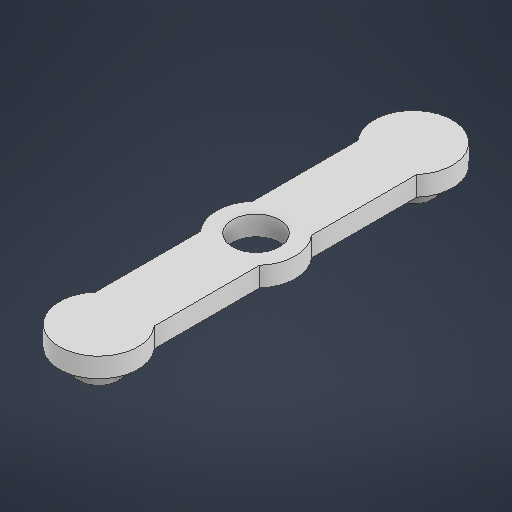
# Autodesk Inventor part: link-split-8ab-2endpins
Saved by Autodesk Inventor 2025.4 (Build 294407000, 407)
## iProperties
Created: 2026-09-15
Part Number: link-split-8ab-2endpins
Material: Generic
Document SubType Name: Modeling
Designer: User
Density: 1 g/cm^3
Appearance: Default
Author: User
Autodesk Inventor part; units mm, degrees
ref_plane "YZ Plane" through (0, 0, 0) normal (1, 0, 0) x (0, 1, 0)
ref_plane "XZ Plane" through (0, 0, 0) normal (0, 1, 0) x (-1, 0, 0)
ref_plane "XY Plane" through (0, 0, 0) normal (0, 0, 1) x (1, 0, 0)
sketch "Sketch1" plane through (0, 0, 0) normal (0, 1, 0) x (-1, 0, 0)
  line L0 (-1.5, -4) -> (1.5, -4)
  line L1 (1.5, -4) -> (1.5, 4)
  line L2 (1.5, 4) -> (-1.5, 4)
  line L3 (-1.5, 4) -> (-1.5, -4)
  line L4 (-1.5, -4) -> (1.5, 4) construction
  line L5 (1.5, -4) -> (-1.5, 4) construction
  circle A0 centre (0, 4) radius 1.2
  circle A1 centre (0, -4) radius 1.2
  circle A2 centre (0, -4) radius 2
  circle A3 centre (0, 4) radius 2
  line L6 (-1.5, 4) -> (1.5, 4)
  line L7 (1.5, 4) -> (1.5, 12)
  line L8 (1.5, 12) -> (-1.5, 12)
  line L9 (-1.5, 12) -> (-1.5, 4)
  circle A4 centre (0, 12) radius 2
  circle A5 centre (0, 12) radius 1.2
  point P0 (0, 0)
  point P1 (-1.5, -2.6771)
  point P2 (1.5, -2.6771)
  point P3 (1.5, 2.6771)
  point P4 (-1.5, 2.6771)
  point P5 (1.5, 10.6771)
  point P6 (-1.5, 10.6771)
  point P7 (-1.5, 5.3229)
  point P8 (1.5, 5.3229)
  dimension "d0" = 3
  dimension "linkPitchA" = 8
  dimension "d3" = 2.4
  dimension "d4" = 4
  dimension "linkPitchB" = 8
  constraints: 20 end point, 6 centre point, 5 midpoint, 5 parallel, 4 equal radius, 3 coincident, 2 horizontal, 2 perpendicular
  measures "d0" distance of L2.end L1.end
  measures "linkPitchA" distance of L1.end L0.end
  measures "d3" diameter of A1
  measures "d4" diameter of A2
  measures "linkPitchB" distance of L7.end L6.end
extrude "Extrusion1" add sketch "Sketch1" along normal blind 1 contours A1 L0 L3 A2 L1 | L0 L1 A2 L3 A1 | A2 L3 A3 L1 | A3 L3 L2 A0 L1 | L1 L7 A3 | L2 A0 L9 A3 L7 | A3 L9 L3 | A3 L9 A4 L7 | A4 L9 L8 A5 L7 | L7 L8 A5 L9 A4
ref_plane "Work Plane2" through (0, 0.5, 0) normal (0, 1, 0) x (1, 0, 0)
sketch "Sketch2" plane through (0, 1, 0) normal (0, 1, 0) x (1, 0, 0)
  line L0 (-1.5, 2.6771) -> (-1.5, -2.6771) projected
  arc A0 (-1.5, -2.6771) -> (-1.5, -5.3229) centre (0, -4) ccw projected
  line L1 (-1.5, -5.3229) -> (-1.5, -10.6771) projected
  arc A1 (-1.5, -10.6771) -> (1.5, -10.6771) centre (0, -12) ccw projected
  line L2 (1.5, -10.6771) -> (1.5, -5.3229) projected
  arc A2 (1.5, -5.3229) -> (1.5, -2.6771) centre (0, -4) ccw projected
  line L3 (1.5, -2.6771) -> (1.5, 2.6771) projected
  arc A3 (1.5, 2.6771) -> (-1.5, 2.6771) centre (0, 4) ccw projected
  circle A4 centre (0, 4) radius 1.2 projected
  circle A5 centre (0, -4) radius 1.2 projected
  circle A6 centre (0, -12) radius 1.2 projected
  circle A7 centre (0, -12) radius 1
  point P0 (0, 0)
  dimension "d22" = 2
  constraints: 1 centre point, 1 coincident
  measures "d22" diameter of A7
extrude "Extrusion2" add sketch "Sketch2" along normal blind 0.5 and the other way blind 1.5 from surface at -0.5 contours A7
sketch "Sketch3" plane through (0, 1, 0) normal (0, 1, 0) x (1, 0, 0)
  line L0 (-1.5, 2.6771) -> (-1.5, -2.6771) projected
  arc A0 (-1.5, -2.6771) -> (-1.5, -5.3229) centre (0, -4) ccw projected
  line L1 (-1.5, -5.3229) -> (-1.5, -10.6771) projected
  arc A1 (-1.5, -10.6771) -> (1.5, -10.6771) centre (0, -12) ccw projected
  line L2 (1.5, -10.6771) -> (1.5, -5.3229) projected
  arc A2 (1.5, -5.3229) -> (1.5, -2.6771) centre (0, -4) ccw projected
  line L3 (1.5, -2.6771) -> (1.5, 2.6771) projected
  arc A3 (1.5, 2.6771) -> (-1.5, 2.6771) centre (0, 4) ccw projected
  circle A4 centre (0, 4) radius 1.2 projected
  circle A5 centre (0, -4) radius 1.2 projected
  circle A6 centre (0, -12) radius 1.2 projected
  circle A7 centre (0, -4) radius 1
  point P0 (0, 0)
  dimension "d23" = 2
  constraints: 1 centre point, 1 coincident
  measures "d23" diameter of A7
extrude "Extrusion3" [suppressed]
sketch "Sketch4" plane through (0, 1, 0) normal (0, 1, 0) x (1, 0, 0)
  line L0 (-1.5, 2.6771) -> (-1.5, -2.6771) projected
  arc A0 (-1.5, -2.6771) -> (-1.5, -5.3229) centre (0, -4) ccw projected
  line L1 (-1.5, -5.3229) -> (-1.5, -10.6771) projected
  arc A1 (-1.5, -10.6771) -> (1.5, -10.6771) centre (0, -12) ccw projected
  line L2 (1.5, -10.6771) -> (1.5, -5.3229) projected
  arc A2 (1.5, -5.3229) -> (1.5, -2.6771) centre (0, -4) ccw projected
  line L3 (1.5, -2.6771) -> (1.5, 2.6771) projected
  arc A3 (1.5, 2.6771) -> (-1.5, 2.6771) centre (0, 4) ccw projected
  circle A4 centre (0, 4) radius 1.2 projected
  circle A5 centre (0, -4) radius 1.2 projected
  circle A6 centre (0, -12) radius 1.2 projected
  circle A7 centre (0, 4) radius 1
  point P0 (0, 0)
  dimension "d24" = 2
  constraints: 1 centre point, 1 coincident
  measures "d24" diameter of A7
extrude "Extrusion4" add sketch "Sketch4" along normal blind 0.5 and the other way blind 1.5 from surface at -0.5 contours A7
sketch "Sketch5" plane through (0, 1, 0) normal (0, 1, 0) x (1, 0, 0)
  line L0 (-1.5, 2.6771) -> (-1.5, -2.6771) projected
  arc A0 (-1.5, -2.6771) -> (-1.5, -5.3229) centre (0, -4) ccw projected
  line L1 (-1.5, -5.3229) -> (-1.5, -10.6771) projected
  arc A1 (-1.5, -10.6771) -> (1.5, -10.6771) centre (0, -12) ccw projected
  line L2 (1.5, -10.6771) -> (1.5, -5.3229) projected
  arc A2 (1.5, -5.3229) -> (1.5, -2.6771) centre (0, -4) ccw projected
  line L3 (1.5, -2.6771) -> (1.5, 2.6771) projected
  arc A3 (1.5, 2.6771) -> (-1.5, 2.6771) centre (0, 4) ccw projected
  circle A4 centre (0, 4) radius 1.2 projected
  circle A5 centre (0, -4) radius 1.2 projected
  circle A6 centre (0, -12) radius 1.2 projected
  point P0 (0, 0)
extrude "Extrusion5" add sketch "Sketch5" against normal blind 1 contours A6
sketch "Sketch6" plane through (0, 1, 0) normal (0, 1, 0) x (1, 0, 0)
  line L0 (-1.5, 2.6771) -> (-1.5, -2.6771) projected
  arc A0 (-1.5, -2.6771) -> (-1.5, -5.3229) centre (0, -4) ccw projected
  line L1 (-1.5, -5.3229) -> (-1.5, -10.6771) projected
  arc A1 (-1.5, -10.6771) -> (1.5, -10.6771) centre (0, -12) ccw projected
  line L2 (1.5, -10.6771) -> (1.5, -5.3229) projected
  arc A2 (1.5, -5.3229) -> (1.5, -2.6771) centre (0, -4) ccw projected
  line L3 (1.5, -2.6771) -> (1.5, 2.6771) projected
  arc A3 (1.5, 2.6771) -> (-1.5, 2.6771) centre (0, 4) ccw projected
  circle A4 centre (0, 4) radius 1.2 projected
  circle A5 centre (0, -4) radius 1.2 projected
  point P0 (0, 0)
extrude "Extrusion6" [suppressed]
sketch "Sketch7" plane through (0, 1, 0) normal (0, 1, 0) x (1, 0, 0)
  line L0 (-1.5, 2.6771) -> (-1.5, -2.6771) projected
  arc A0 (-1.5, -2.6771) -> (-1.5, -5.3229) centre (0, -4) ccw projected
  line L1 (-1.5, -5.3229) -> (-1.5, -10.6771) projected
  arc A1 (-1.5, -10.6771) -> (1.5, -10.6771) centre (0, -12) ccw projected
  line L2 (1.5, -10.6771) -> (1.5, -5.3229) projected
  arc A2 (1.5, -5.3229) -> (1.5, -2.6771) centre (0, -4) ccw projected
  line L3 (1.5, -2.6771) -> (1.5, 2.6771) projected
  arc A3 (1.5, 2.6771) -> (-1.5, 2.6771) centre (0, 4) ccw projected
  circle A4 centre (0, 4) radius 1.2 projected
  point P0 (0, 0)
extrude "Extrusion7" add sketch "Sketch7" against normal blind 1 contours A4
body "Solid1"
